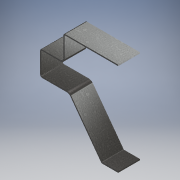
# Autodesk Inventor part: CAR INTERNAL PLATE
Saved by Autodesk Inventor 2017 (Build 210142000, 142)
## iProperties
Part Number: CAR INTERNAL PLATE
Material: Genérico
Document SubType Name: Modeling
Designer: Cristian
Density: 1 g/cm^3
Appearance: Valor por defecto
Author: Cristian
Autodesk Inventor part; units mm, degrees
ref_plane "YZ Plane" through (0, 0, 0) normal (1, 0, 0) x (0, 1, 0)
ref_plane "XZ Plane" through (0, 0, 0) normal (0, 1, 0) x (-1, 0, 0)
ref_plane "XY Plane" through (0, 0, 0) normal (0, 0, 1) x (1, 0, 0)
sketch "Boceto1" plane through (0, 0, 0) normal (0, 1, 0) x (-1, 0, 0)
  line L0 (0, 0) -> (273.05, 0)
  line L1 (273.05, 0) -> (273.05, -101.6)
  line L2 (273.05, -101.6) -> (368.3, -101.6)
  line L3 (368.3, -101.6) -> (368.3, -212.725)
  line L4 (0, 0) -> (0, -393.7)
  line L5 (0, -393.7) -> (114.3, -393.7)
  line L6 (368.3, -212.725) -> (247.65, -212.725)
  line L7 (247.65, -212.725) -> (114.3, -393.7)
  dimension "d0" = 273.05
  dimension "d1" = 101.6
  dimension "d2" = 95.25
  dimension "d3" = 111.125
  dimension "d4" = 393.7
  dimension "d50" = 114.3
  dimension "d51" = 133.35
  constraints: 16 end point, 3 horizontal, 2 perpendicular, 2 vertical
  measures "d0" distance of L0.start L0.end
  measures "d1" distance of L0.end L1.end
  measures "d2" distance of L1.end L2.end
  measures "d3" distance of L2.end L3.end
  measures "d4" distance of L0.start L4.end
  measures "d50" distance of L4.end L5.end
  measures "d51" horizontal distance of L5.end L6.end
extrude "Extrusión1" add sketch "Boceto1" along normal blind 5
fillet "Empalme1" radius 12.7 7 edges at (-368.3, 2.5, -101.6) (-273.05, 2.5, 0) (-368.3, 2.5, -212.725) (-247.65, 2.5, -212.725) (-114.3, 2.5, -393.7) (0, 2.5, -393.7) (0, 2.5, 0)
fillet "Empalme2" radius 6.35 1 edges at (-273.05, 2.5, -101.6)
sketch "Boceto2" plane through (0, 5, 0) normal (0, 1, 0) x (1, 0, 0)
  line L0 (-349.25, 119.0625) -> (-273.05, 119.0625)
  line L1 (-273.05, 119.0625) -> (-273.05, 195.2625)
  line L2 (-273.05, 195.2625) -> (-349.25, 195.2625)
  line L3 (-349.25, 195.2625) -> (-349.25, 119.0625)
  line L4 (-368.3, 200.025) -> (-368.3, 114.3) projected
  line L5 (-254.0674, 212.725) -> (-355.6, 212.725) projected
  line L6 (-355.6, 101.6) -> (-279.4, 101.6) projected
  line L7 (-260.35, 0) -> (-12.7, 0) projected
  line L8 (-43.6563, 0) -> (-38.1, 0)
  line L9 (-38.1, 0) -> (-38.1, 6.35)
  line L10 (-38.1, 6.35) -> (-43.6562, 6.35)
  line L11 (-43.6562, 6.35) -> (-43.6563, 0)
  line L12 (-12.7, 393.7) -> (-107.8826, 393.7) projected
  line L13 (0, 12.7) -> (0, 381) projected
  circle A0 centre (-98.0281, 104.775) radius 4.3656
  circle A1 centre (-59.9281, 104.775) radius 4.3656
  circle A2 centre (-98.0281, 288.925) radius 4.3656
  circle A3 centre (-59.9281, 288.925) radius 4.3656
  line L14 (-123.825, 158.75) -> (-47.625, 158.75)
  line L15 (-47.625, 158.75) -> (-47.625, 234.95)
  line L16 (-47.625, 234.95) -> (-123.825, 234.95)
  line L17 (-123.825, 234.95) -> (-123.825, 158.75)
  circle A4 centre (-42.6641, 365.125) radius 5
  circle A5 centre (-42.6641, 28.575) radius 5
  line L18 (-107.8826, 393.7) -> (-12.7, 393.7) projected
  line L19 (-43.6563, 393.7) -> (-38.1, 393.7)
  line L20 (-38.1, 393.7) -> (-38.1, 387.35)
  line L21 (-38.1, 387.35) -> (-43.6563, 387.35)
  line L22 (-43.6563, 387.35) -> (-43.6563, 393.7)
  line L23 (-42.8625, 127) -> (-38.1, 127)
  line L24 (-38.1, 127) -> (-38.1, 140.0969)
  line L25 (-38.1, 140.0969) -> (-42.8625, 140.0969)
  line L26 (-42.8625, 140.0969) -> (-42.8625, 127)
  line L27 (-42.8625, 190.5) -> (-38.1, 190.5)
  line L28 (-38.1, 190.5) -> (-38.1, 203.5969)
  line L29 (-38.1, 203.5969) -> (-42.8625, 203.5969)
  line L30 (-42.8625, 203.5969) -> (-42.8625, 190.5)
  line L31 (-42.8625, 254) -> (-38.1, 254)
  line L32 (-38.1, 254) -> (-38.1, 267.0969)
  line L33 (-38.1, 267.0969) -> (-42.8625, 267.0969)
  line L34 (-42.8625, 267.0969) -> (-42.8625, 254)
  point P0 (0, 0)
  dimension "d11" = 76.2
  dimension "d17" = 17.4625
  dimension "d18" = 19.05
  dimension "d19" = 76.2
  dimension "d20" = 5.5563
  dimension "d22" = 6.35
  dimension "d24" = 38.1
  dimension "d27" = 8.7312
  dimension "d38" = 76.2
  dimension "d39" = 76.2
  dimension "d40" = 158.75
  dimension "d42" = 10
  dimension "d43" = 28.575
  dimension "d44" = 42.6641
  dimension "d47" = 10
  dimension "d52" = 38.1
  dimension "d53" = 5.5563
  dimension "d54" = 6.35
  dimension "d55" = 47.625
  dimension "d56" = 8.7312
  dimension "d57" = 98.0281
  dimension "d58" = 38.1
  dimension "d59" = 53.975
  dimension "d60" = 53.975
  dimension "d61" = 184.15
  dimension "d62" = 184.15
  dimension "d63" = 38.1
  dimension "d64" = 8.7312
  dimension "d65" = 8.7312
  dimension "d66" = 98.0281
  dimension "d67" = 42.6641
  dimension "d68" = 28.575
  dimension "d69" = 4.7625
  dimension "d70" = 4.7625
  dimension "d71" = 4.7625
  dimension "d72" = 13.0969
  dimension "d73" = 13.0969
  dimension "d74" = 13.0969
  dimension "d75" = 38.1
  dimension "d80" = 63.5
  dimension "d81" = 63.5
  dimension "d82" = 127
  constraints: 56 end point, 14 parallel, 7 horizontal, 7 perpendicular, 6 centre point, 3 point on line, 1 collinear
  measures "d11" distance of L2.end L0.start
  measures "d17" distance between parallel lines of L0 L6
  measures "d18" distance between parallel lines of L3 L4
  measures "d19" distance of L1.end L2.end
  measures "d20" distance between parallel lines of L9 L11
  measures "d22" distance of L10.end L8.start
  measures "d24" distance between parallel lines of L13 L9
  measures "d27" diameter of A1
  measures "d38" distance of L16.end L14.start
  measures "d39" distance between parallel lines of L15 L17
  measures "d40" distance between parallel lines of L7 L14
  measures "d42" diameter of A4
  measures "d43" distance from line of L12 A4.centre
  measures "d44" distance from line of L13 A4.centre
  measures "d47" diameter of A5
  measures "d52" distance between parallel lines of L13 L20
  measures "d53" distance between parallel lines of L20 L22
  measures "d54" distance of L21.end L19.start
  measures "d55" distance between parallel lines of L13 L15
  measures "d56" diameter of A0
  measures "d57" distance from line of L13 A0.centre
  measures "d58" distance of A1.centre A0.centre
  measures "d59" distance from line of L14 A0.centre
  measures "d60" distance from line of L14 A1.centre
  measures "d61" distance of A2.centre A0.centre
  measures "d62" distance of A1.centre A3.centre
  measures "d63" distance of A3.centre A2.centre
  measures "d64" diameter of A2
  measures "d65" diameter of A3
  measures "d66" distance from line of L13 A2.centre
  measures "d67" distance from line of L13 A5.centre
  measures "d68" distance from line of L7 A5.centre
  measures "d69" distance of L25.end L24.end
  measures "d70" distance of L29.end L28.end
  measures "d71" distance between parallel lines of L32 L34
  measures "d72" distance between parallel lines of L25 L23
  measures "d73" distance of L27.end L28.end
  measures "d74" distance of L31.end L32.end
  measures "d75" distance between parallel lines of L13 L24
  measures "d80" distance between parallel lines of L27 L23
  measures "d81" distance between parallel lines of L31 L27
  measures "d82" distance between parallel lines of L7 L23
extrude "Extrusión2" cut sketch "Boceto2" against normal up to next
fillet "Empalme3" radius 3.5719 8 edges at (-349.25, 2.5, -119.0625) (-123.825, 2.5, -158.75) (-349.25, 2.5, -195.2625) (-123.825, 2.5, -234.95) (-273.05, 2.5, -195.2625) (-47.625, 2.5, -234.95) (-273.05, 2.5, -119.0625) (-47.625, 2.5, -158.75)
sketch "Boceto3" plane through (0, 5, 0) normal (0, 1, 0) x (1, 0, 0)
  line L0 (0, 12.7) -> (0, 381) projected
  line L1 (0, 381) -> (0, 12.7) projected
  line L2 (0, 196.85) -> (-12.7, 196.85)
  line L3 (0, 196.85) -> (0, 219.075)
  line L4 (0, 196.85) -> (0, 174.625)
  arc A0 (0, 219.075) -> (0, 174.625) centre (13.0969, 196.85) ccw
  point P0 (0, 0)
  dimension "d86" = 12.7
  dimension "d87" = 22.225
  dimension "d88" = 22.225
  constraints: 6 end point, 3 point on circle, 2 point on line, 1 centre point, 1 horizontal, 1 midpoint
  measures "d86" distance of L2.start L2.end
  measures "d87" distance of L2.start L3.end
  measures "d88" distance of L2.start L4.end
extrude "Extrusión3" cut sketch "Boceto3" against normal up to next
fillet "Empalme4" radius 4.7625 2 edges at (0, 2.5, -219.075) (0, 2.5, -174.625)
sketch "Boceto4" plane through (0, 0, 0) normal (0, -1, 0) x (1, 0, 0)
  line L0 (-43.6562, -5) -> (-260.35, -5)
  line L1 (-268.05, -12.7) -> (-268.05, -95.25)
  line L2 (-279.4, -106.6) -> (-355.6, -106.6)
  line L3 (-363.3, -114.3) -> (-363.3, -200.025)
  line L4 (-355.6, -207.725) -> (-254.0138, -207.725)
  line L5 (-239.693, -214.9673) -> (-114.1714, -385.5509)
  line L6 (-107.9443, -388.7) -> (-43.6563, -388.7)
  line L7 (-107.8826, -393.7) -> (-43.6563, -393.7) projected
  line L8 (-118.1068, -388.5336) -> (-243.8432, -217.8914) projected
  line L9 (-355.6, -212.725) -> (-254.0674, -212.725) projected
  line L10 (-368.3, -200.025) -> (-368.3, -114.3) projected
  line L11 (-43.6563, -387.35) -> (-43.6563, -393.7) projected
  line L12 (-355.6, -101.6) -> (-279.4, -101.6) projected
  line L13 (-273.05, -95.25) -> (-273.05, -12.7) projected
  line L14 (-260.35, 0) -> (-43.6563, 0) projected
  line L15 (-43.6563, 0) -> (-43.6562, -6.35) projected
  arc A0 (-363.3, -200.025) -> (-355.6, -207.725) centre (-355.6, -200.025) ccw
  line L16 (-368.3, -114.3) -> (-368.3, -200.025) projected
  arc A1 (-355.6, -106.6) -> (-363.3, -114.3) centre (-355.6, -114.3) ccw
  arc A2 (-260.35, -5) -> (-268.05, -12.7) centre (-260.35, -12.7) ccw
  arc A3 (-279.4, -106.6) -> (-268.05, -95.25) centre (-279.4, -95.25) ccw
  line L17 (-273.05, -12.7) -> (-273.05, -95.25) projected
  line L18 (-174.9103, -311.4431) -> (-170.8831, -308.4798)
  arc A4 (-239.693, -214.9673) -> (-254.0138, -207.725) centre (-254.0138, -225.505) ccw
  arc A5 (-114.1714, -385.5509) -> (-107.9443, -388.7) centre (-107.9443, -380.9688) ccw
  line L19 (-43.6563, -383.7) -> (-107.9443, -383.7)
  arc A6 (-110.1442, -382.5875) -> (-107.9443, -383.7) centre (-107.9443, -380.9688) ccw
  line L20 (-110.1442, -382.5875) -> (-235.6658, -212.0039)
  arc A7 (-235.6658, -212.0039) -> (-254.0138, -202.725) centre (-254.0138, -225.505) ccw
  line L21 (-254.0138, -202.725) -> (-355.6, -202.725)
  arc A8 (-358.3, -200.025) -> (-355.6, -202.725) centre (-355.6, -200.025) ccw
  line L22 (-358.3, -200.025) -> (-358.3, -114.3)
  arc A9 (-355.6, -111.6) -> (-358.3, -114.3) centre (-355.6, -114.3) ccw
  line L23 (-355.6, -111.6) -> (-279.4, -111.6)
  arc A10 (-279.4, -111.6) -> (-263.05, -95.25) centre (-279.4, -95.25) ccw
  line L24 (-263.05, -95.25) -> (-263.05, -12.7)
  arc A11 (-260.35, -10) -> (-263.05, -12.7) centre (-260.35, -12.7) ccw
  line L25 (-260.35, -10) -> (-43.6562, -10)
  line L26 (-43.6563, -383.7) -> (-43.6563, -388.7)
  line L27 (-43.6562, -5) -> (-43.6562, -10)
  line L28 (-43.6562, -6.35) -> (-43.6563, 0) projected
  point P0 (0, 0)
  dimension "d92" = 5
  dimension "d95" = 5
  dimension "d96" = 5
  dimension "d99" = 5
  dimension "d100" = 5
  dimension "d101" = 5
  dimension "d102" = 0
  dimension "d105" = 0
  dimension "d109" = 0
  dimension "d110" = 5
  dimension "d115" = 17.78
  dimension "d117" = 5
  dimension "d118" = 7.7312
  constraints: 34 end point, 24 point on circle, 12 centre point, 12 tangent, 9 perpendicular, 4 parallel, 2 point on line, 1 collinear, 1 horizontal, 1 vertical, 13 other
  measures "d92" distance between parallel lines of L7 L6
  measures "d95" distance between parallel lines of L9 L4
  measures "d96" distance between parallel lines of L10 L3
  measures "d99" distance between parallel lines of L12 L2
  measures "d100" distance between parallel lines of L13 L1
  measures "d101" distance between parallel lines of L14 L0
  measures "d102" distance from line of L15 L0.start
  measures "d105" vertical distance of L10.start L3.end
  measures "d109" vertical distance of L13.start L1.end
  measures "d110" distance of L18.start L18.end
  measures "d115" radius of A4
  measures "d117" distance between parallel lines of L5 L20
  measures "d118" radius of A5
extrude "Extrusión4" add sketch "Boceto4" along normal blind 88.9
sketch "Boceto5" plane through (0, 5, 0) normal (0, 1, 0) x (1, 0, 0)
  line L0 (88.3096, -76.4471) -> (-485.0439, -76.4471)
  line L1 (-485.0439, -76.4471) -> (-485.0439, 517.9952)
  line L2 (-485.0439, 517.9952) -> (88.3096, 517.9952)
  line L3 (88.3096, 517.9952) -> (88.3096, -76.4471)
  point P0 (0, 0)
  constraints: 8 end point, 2 parallel, 1 horizontal, 1 perpendicular
extrude "Extrusión5" cut sketch "Boceto5" against normal up to surface (5 mm away)
equation "\"d42\" = UBD"
equation "\"d47\" = UBD"
equation "\"LM\" = 76.2"
equation "\"UBD\" = 10"
